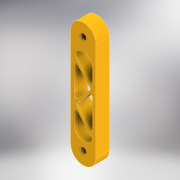
# Autodesk Inventor part: CodoTrasero
Saved by Autodesk Inventor 2021 (Build 250183000, 183)
## iProperties
Created: 2024-02-25
Part Number: CodoTrasero
Material: PLA
Document SubType Name: Modeling
Designer: Martin
Mass: 70.7951 g
Surface Area: 214.305 cm^2
Volume: 55.7442 cm^3
Density: 1.27 g/cm^3
Appearance: PLA
Author: Martin
Autodesk Inventor part; units mm, degrees
ref_plane "YZ Plane" through (0, 0, 0) normal (1, 0, 0) x (0, 1, 0)
ref_plane "XZ Plane" through (0, 0, 0) normal (0, 1, 0) x (-1, 0, 0)
ref_plane "XY Plane" through (0, 0, 0) normal (0, 0, 1) x (1, 0, 0)
sketch "Sketch1" plane through (0, 0, 0) normal (0, 0, 1) x (1, 0, 0)
  line L0 (0, 66) -> (0, -66) construction
  line L1 (-17, 66) -> (-17, -66)
  line L2 (17, -66) -> (17, 66)
  arc A0 (17, 66) -> (-17, 66) centre (0, 66) ccw
  arc A1 (-17, -66) -> (17, -66) centre (0, -66) ccw
  circle A2 centre (0, -66) radius 1.1
  circle A3 centre (0, 66) radius 11.1
  point P0 (0, 0)
  dimension "d0" = 66
  dimension "d1" = 34
  dimension "d2" = 2.2
  dimension "d3" = 22.2
  dimension "d40" = 17
  constraints: 8 end point, 4 centre point, 4 point on circle, 4 tangent, 2 coincident, 1 midpoint, 1 parallel, 1 vertical
  measures "d0" distance of point (0, 0) L0.end
  measures "d1" diameter of A1
  measures "d2" diameter of A2
  measures "d3" diameter of A3
  measures "d40" radius of A0
extrude "Extrusion1" add sketch "Sketch1" along normal blind 8
sketch "Sketch2" plane through (0, 0, 8) normal (0, 0, 1) x (1, 0, 0)
  arc A0 (-17, -66) -> (17, -66) centre (0, -66) ccw projected
  line L0 (17, -66) -> (17, 66) projected
  arc A1 (17, 66) -> (-17, 66) centre (0, 66) ccw projected
  line L1 (-17, 66) -> (-17, -66) projected
  circle A2 centre (0, 66) radius 11.1 projected
  circle A3 centre (0, -66) radius 1.1 projected
  circle A4 centre (0, -66) radius 4.1
  circle A5 centre (0, 66) radius 4.1
  point P0 (0, 0)
  dimension "d6" = 8.2
  dimension "d12" = 8.2
  constraints: 2 centre point, 2 coincident
  measures "d6" diameter of A4
  measures "d12" diameter of A5
extrude "Extrusion2" add sketch "Sketch2" along normal blind 10 contours L1 A1 L0 A0 | A2
sketch "Sketch3" plane through (0, 0, 18) normal (0, 0, 1) x (1, 0, 0)
  line L0 (17, -66) -> (17, 66) projected
  arc A0 (17, 66) -> (-17, 66) centre (0, 66) ccw projected
  line L1 (-17, 66) -> (-17, -66) projected
  arc A1 (-17, -66) -> (17, -66) centre (0, -66) ccw projected
  circle A2 centre (0, -66) radius 4.1 projected
  line L2 (0, 49) -> (0, -56) construction
  line L3 (-12, 37) -> (-12, -44)
  line L4 (12, -44) -> (12, 37)
  arc A3 (12, 37) -> (-12, 37) centre (0, 37) ccw
  arc A4 (-12, -44) -> (12, -44) centre (0, -44) ccw
  line L5 (-12, -44) -> (-12, -17)
  line L6 (12, 37) -> (12, 10)
  line L7 (12, -44) -> (-12, -17)
  line L8 (-12, -17) -> (12, 10)
  line L9 (12, 10) -> (-12, 37)
  line L10 (13.1211, 10.9965) -> (-11.8222, 39.0578)
  line L11 (10.8789, 9.0035) -> (-13.1211, 36.0035)
  line L12 (-13.1211, -16.0035) -> (10.8789, 10.9965)
  line L13 (11.8222, -46.0578) -> (-13.1211, -17.9965)
  line L14 (13.1211, -43.0035) -> (-10.8789, -16.0035)
  line L15 (-10.8789, -17.9965) -> (13.1211, 9.0035)
  point P0 (0, -3.5)
  point P1 (-12, -19.2578)
  point P2 (12, 7.7422)
  point P3 (-9.9931, -17)
  point P4 (12, -41.7422)
  point P5 (-12, -14.7422)
  point P6 (9.9931, 10)
  point P7 (-12, 34.7422)
  point P8 (12, 12.2578)
  dimension "d47" = 105
  dimension "d48" = 24
  dimension "d49" = 27
  dimension "d50" = 27
  dimension "d51" = 1.5
  dimension "d52" = 1.5
  dimension "d53" = 1.5
  dimension "d54" = 1.5
  dimension "d55" = 1.5
  dimension "d56" = 1.5
  constraints: 30 end point, 8 point on circle, 7 parallel, 4 point on line, 4 tangent, 2 centre point, 1 midpoint, 1 vertical
  measures "d47" distance of L2.start L2.end
  measures "d48" diameter of A4
  measures "d49" distance of L3.end L5.end
  measures "d50" distance of L4.end L6.end
  measures "d51" distance between parallel lines of L9 L10
  measures "d52" distance between parallel lines of L9 L11
  measures "d53" distance between parallel lines of L8 L12
  measures "d54" distance between parallel lines of L7 L13
  measures "d55" distance between parallel lines of L7 L14
  measures "d56" distance between parallel lines of L8 L15
extrude "Extrusion3" cut sketch "Sketch3" against normal up to next contours L11 L12 L3 | A3 L4 L10 | L4 L14 L15 | L13 A4 L3
sketch "Sketch6" plane through (0, -66, 8) normal (0, 0, 1) x (1, 0, 0)
  circle A0 centre (0, 0) radius 4.1 projected
  circle A1 centre (0, 0) radius 1.1 projected
  point P0 (0, 66)
extrude "Extrusion6" cut sketch "Sketch6" against normal up to next
fillet "Fillet3" radius 2 10 edges at (-12, 34.7422, 9) (12, 12.2578, 9) (9.9931, 10, 9) (12, 7.7422, 9) (-12, -14.7422, 9) (-9.9931, -17, 9) (-12, -19.2578, 9) (12, -41.7422, 9) (11.8222, -46.0578, 9) (-11.8222, 39.0578, 9)
equation "\"d12\" = d6"
equation "\"d50\" = d49"
body "Solid1"
